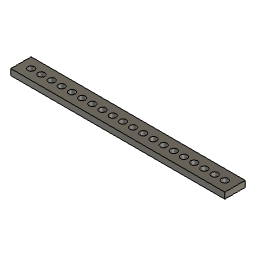
Quadrupedalism_LegsJoint (Autodesk Fusion 360 design; units mm, degrees)
Autodesk Fusion 360 part; units mm, degrees
sketch "Sketch1" plane through (0, 0, 0) normal (0, 0, 1) x (1, 0, 0)
  circle A0 centre (0, 0) radius 1.6
  line L0 (-5, 5) -> (100, 5)
  line L1 (100, 5) -> (100, -5)
  line L2 (100, -5) -> (-5, -5)
  line L3 (-5, -5) -> (-5, 5)
  line L4 (-5, 0) -> (100, 0) construction
  circle A1 centre (5, 0) radius 1.6
  circle A2 centre (10, 0) radius 1.6
  circle A3 centre (15, 0) radius 1.6
  circle A4 centre (20, 0) radius 1.6
  circle A5 centre (25, 0) radius 1.6
  circle A6 centre (30, 0) radius 1.6
  circle A7 centre (35, 0) radius 1.6
  circle A8 centre (40, 0) radius 1.6
  circle A9 centre (45, 0) radius 1.6
  circle A10 centre (50, 0) radius 1.6
  circle A11 centre (55, 0) radius 1.6
  circle A12 centre (60, 0) radius 1.6
  circle A13 centre (65, 0) radius 1.6
  circle A14 centre (70, 0) radius 1.6
  circle A15 centre (75, 0) radius 1.6
  circle A16 centre (80, 0) radius 1.6
  circle A17 centre (85, 0) radius 1.6
  circle A18 centre (90, 0) radius 1.6
  circle A19 centre (95, 0) radius 1.6
  dimension "d56" = 3.2
  dimension "d57" = 5
  dimension "d58" = 10
  dimension "d59" = 105
  dimension "d62" = 5
  dimension "d63" = 0
  constraint coincident A0.centre origin
  constraint horizontal L0
  constraint vertical L1
  constraint horizontal L2
  constraint vertical L3
  constraint midpoint L3 L4.start
  constraint midpoint L1 L4.end
  constraint coincident A0.centre L4
  measures "d56" diameter of A0
  measures "d57" distance of A0.centre L3
  measures "d58" distance of L0.start L2.end
  measures "d59" distance of L0.start L0.end
extrude "Extrude1" add sketch "Sketch1" along normal blind 3
move_body "Move1" [suppressed]
equation "d56 = HoleDiameter"
equation "d57 = HoleSpacing"
equation "d58 = LegWidth"
equation "d59 = LegsJointLength"
equation "d60 = LegsJointLength / HoleSpacing - 1"
equation "d62 = HoleSpacing"
equation "d64 = Thickness"
equation "HoleDiameter = 3.2 mm"
equation "Thickness = 3 mm"
equation "HoleSpacing = 5 mm"
equation "LegWidth = 10 mm"
equation "LegsJointLength = 105 mm"
